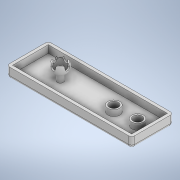
# Autodesk Inventor part: Base
Saved by Autodesk Inventor 2021 (Build 250183000, 183)
## iProperties
Created: 2021-03-30
Part Number: Base
Material: Generic
Document SubType Name: Modeling
Designer: eng1-177
Density: 1 g/cm^3
Appearance: Default
Author: eng1-177
Autodesk Inventor part; units mm, degrees
ref_plane "YZ Plane" through (0, 0, 0) normal (1, 0, 0) x (0, 1, 0)
ref_plane "XZ Plane" through (0, 0, 0) normal (0, 1, 0) x (-1, 0, 0)
ref_plane "XY Plane" through (0, 0, 0) normal (0, 0, 1) x (1, 0, 0)
sketch "Sketch1" plane through (0, 0, 0) normal (0, 0, 1) x (1, 0, 0)
  line L0 (0, 0) -> (5, 0)
  line L1 (5, 0) -> (5, 10)
  line L2 (5, 10) -> (0, 10)
  line L3 (0, 10) -> (0, 0)
  arc A0 (0, 10) -> (0, 35) centre (0, 22.5) ccw
  arc A1 (0, 12.5) -> (8.9476, 26.9654) centre (0, 22.5) ccw
  line L4 (0, 12.5) -> (0, 10)
  line L5 (5, 10) -> (5, 11.0436)
  line L6 (8.9476, 28.1438) -> (11.1534, 28.1438)
  line L7 (8.9476, 28.1438) -> (8.9476, 26.9654)
  dimension "d0" = 5
  dimension "d1" = 10
  dimension "d2" = 25
  dimension "d3" = 20
  constraints: 16 end point, 6 point on circle, 3 parallel, 3 perpendicular, 2 centre point, 1 coincident, 1 horizontal, 1 tangent, 1 vertical
  measures "d0" distance of L2.end L1.end
  measures "d1" distance of L1.end L0.end
  measures "d2" distance of L2.end A0.end
  measures "d3" diameter of A1
revolve "Revolution1" add sketch "Sketch1" angle 360 about axis through (0, 10, 0) along (0, -1, 0)
sketch "Sketch2" plane through (0, 28.1438, 0) normal (0, 1, 0) x (1, 0, 0)
  line L0 (3.75, 3.75) -> (3.75, 15)
  line L1 (3.75, 15) -> (0, 15)
  line L2 (-3.75, 3.75) -> (-3.75, 15)
  line L3 (-3.75, 15) -> (0, 15)
  line L4 (3.75, -3.75) -> (3.75, -15.018)
  line L5 (3.75, -15.018) -> (-3.75, -15.018)
  line L6 (-3.75, -15.018) -> (-3.75, -3.75)
  line L7 (-15.3562, 0) -> (-15.3562, 3.75)
  line L8 (-15.3562, 3.75) -> (-3.75, 3.75)
  line L9 (-15.3562, 0) -> (-15.3562, -3.75)
  line L10 (-15.3562, -3.75) -> (-3.75, -3.75)
  line L11 (3.75, 3.75) -> (17.3857, 3.75)
  line L12 (17.3857, 3.75) -> (17.3857, -3.75)
  line L13 (17.3857, -3.75) -> (3.75, -3.75)
  point P0 (0, 0)
  constraints: 28 end point, 2 parallel, 2 point on line, 1 horizontal, 1 perpendicular
extrude "Extrusion1" cut sketch "Sketch2" against normal blind 7.5
fillet "Fillet1" radius 3.75 8 edges at (-3.75, 20.6438, 10.4307) (-10.4307, 20.6438, -3.75) (-3.75, 20.6438, -10.4307) (10.4307, 20.6438, -3.75) (10.4307, 20.6438, 3.75) (3.75, 20.6438, 10.4307) (-10.4307, 20.6438, 3.75) (3.75, 20.6438, -10.4307)
sketch "Sketch3" plane through (0, 0, 0) normal (0, -1, 0) x (1, 0, 0)
  line L0 (0, 0) -> (-50, 0)
  line L1 (-50, 0) -> (-50, 30)
  line L2 (-50, 30) -> (0, 30)
  line L3 (0, 30) -> (0, 0)
  line L4 (0, 0) -> (-50, 0)
  line L5 (-50, 0) -> (-50, -30)
  line L6 (-50, -30) -> (0, -30)
  line L7 (0, -30) -> (0, 0)
  dimension "d13" = 50
  dimension "d14" = 30
  dimension "d15" = 50
  dimension "d16" = 30
  constraints: 16 end point, 4 parallel, 2 horizontal, 2 perpendicular
  measures "d13" distance of L1.end L2.end
  measures "d14" distance of L0.end L1.end
  measures "d15" distance of L6.end L5.end
  measures "d16" distance of L5.end L4.end
extrude "Extrusion2" add sketch "Sketch3" along normal blind 5
sketch "Sketch4" plane through (-50, 0, 30) normal (0, 0, 1) x (1, 0, 0)
  line L0 (50, -5) -> (0, -5) projected
  line L1 (0, -5) -> (50, -5)
  line L2 (50, -5) -> (50, 12.5)
  line L3 (50, 12.5) -> (0, 12.5)
  line L4 (0, 12.5) -> (0, -5)
  point P0 (50, 0)
  dimension "d19" = 50
  dimension "d20" = 17.5
  constraints: 8 end point, 2 parallel, 1 horizontal, 1 perpendicular
  measures "d19" distance of L3.end L2.end
  measures "d20" distance of L2.end L1.end
extrude "Extrusion3" add sketch "Sketch4" along normal blind 5
sketch "Sketch5" plane through (0, 0, -30) normal (0, 0, -1) x (-1, 0, 0)
  line L0 (50, -5) -> (0, -5) projected
  line L1 (0, -5) -> (50, -5)
  line L2 (50, -5) -> (50, 12.5)
  line L3 (50, 12.5) -> (0, 12.5)
  line L4 (0, 12.5) -> (0, -5)
  point P0 (0, 0)
  dimension "d23" = 50
  dimension "d24" = 17.5
  constraints: 8 end point, 2 parallel, 1 horizontal, 1 perpendicular
  measures "d23" distance of L3.end L2.end
  measures "d24" distance of L2.end L1.end
extrude "Extrusion4" add sketch "Sketch5" along normal blind 5
sketch "Sketch6" plane through (-50, 0, 30) normal (-1, 0, 0) x (0, 0, 1)
  line L0 (-60, 12.5) -> (-65, 12.5) projected
  line L1 (5, -5) -> (5, 12.5) projected
  line L2 (-65, 12.5) -> (5, 12.5)
  line L3 (5, 12.5) -> (5, -5)
  line L4 (5, -5) -> (-65, -5)
  line L5 (-65, -5) -> (-65, 12.5)
  point P0 (-30, 0)
  constraints: 8 end point, 2 parallel, 1 horizontal, 1 perpendicular
extrude "Extrusion5" add sketch "Sketch6" along normal blind 5
sketch "Sketch7" plane through (0, 0, 5) normal (1, 0, 0) x (0, 0, -1)
  line L0 (-25, 12.5) -> (-25, 0) projected
  line L1 (-25, 0) -> (-25, 12.5)
  line L2 (-30, -5) -> (-30, 12.5) projected
  line L3 (-25, 12.5) -> (-30, 12.5)
  line L4 (-30, -5) -> (40, -5) projected
  line L5 (-30, 12.5) -> (-30, -5)
  line L6 (-30, -5) -> (40, -5)
  line L7 (40, 12.5) -> (40, -5) projected
  line L8 (40, -5) -> (40, 12.5)
  line L9 (35, 12.5) -> (35, 0) projected
  line L10 (40, 12.5) -> (35, 12.5)
  line L11 (35, 12.5) -> (35, 0)
  line L12 (0, 0) -> (-25, 0) projected
  line L13 (35, 0) -> (-25, 0)
  point P0 (5, 0)
  constraints: 16 end point, 5 collinear, 3 perpendicular
extrude "Extrusion6" add sketch "Sketch7" along normal blind 155
sketch "Sketch8" plane through (155, 0, 5) normal (1, 0, 0) x (0, 0, -1)
  line L0 (-25, 12.5) -> (-25, 0) projected
  line L1 (-25, 0) -> (35, 0) projected
  line L2 (-25, 12.5) -> (35, 12.5)
  line L3 (35, 12.5) -> (35, 0)
  line L4 (35, 0) -> (-25, 0)
  line L5 (-25, 0) -> (-25, 12.5)
  point P0 (5, 0)
  constraints: 8 end point, 2 parallel, 1 horizontal, 1 perpendicular
extrude "Extrusion7" add sketch "Sketch8" against normal blind 5
sketch "Sketch9" plane through (0, 0, 0) normal (0, 1, 0) x (1, 0, 0)
  line L0 (-50, 30) -> (150, 30) projected
  line L1 (-50, -30) -> (150, -30) projected
  line L2 (150, 30) -> (70, 30)
  line L3 (70, -30) -> (150, -30)
  line L4 (150, -30) -> (150, 30)
  line L5 (70, -30) -> (110, -30)
  line L6 (110, 30) -> (70, 30)
  line L7 (70, 30) -> (70, -30)
  circle A0 centre (90, 0) radius 10
  line L8 (110, 30) -> (130, 30)
  line L9 (130, -30) -> (110, -30)
  line L10 (110, -30) -> (110, 30)
  circle A1 centre (130, 0) radius 10
  point P0 (0, 0)
  dimension "d34" = 20
  constraints: 18 end point, 3 horizontal, 3 parallel, 2 centre point, 2 point on line, 1 midpoint
  measures "d34" diameter of A0
extrude "Extrusion8" add sketch "Sketch9" along normal blind 10 contours A0 | A1
sketch "Sketch10" plane through (90, 10, 0) normal (0, 1, 0) x (1, 0, 0)
  circle A0 centre (0, 0) radius 7.5
  circle A1 centre (40, 0) radius 10 projected
  circle A2 centre (40, 0) radius 7.5
  point P0 (-90, 0)
  dimension "d38" = 15
  constraints: 2 centre point, 1 coincident
  measures "d38" diameter of A0
extrude "Extrusion9" cut sketch "Sketch10" against normal blind 10 contours A0 | A2
fillet "Fillet2" radius 5 4 edges at (-55, 3.75, 35) (155, 3.75, 35) (155, 3.75, -35) (-55, 3.75, -35)
fillet "Fillet3" radius 5 8 edges at (153.5355, -5, -33.5355) (50, -5, -35) (-53.5355, -5, -33.5355) (-55, -5, 0) (-53.5355, -5, 33.5355) (50, -5, 35) (153.5355, -5, 33.5355) (155, -5, 0)
body "Solid1"
